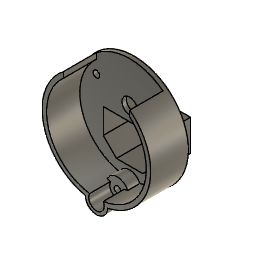
ElementCover v7 (Autodesk Fusion 360 design; units mm, degrees)
Autodesk Fusion 360 part; units mm, degrees
sketch "Sketch1" plane through (0, 0, 0) normal (0, 1, 0) x (1, 0, 0)
  circle A0 centre (-4.2105, -0.0551) radius 22.5
  circle A1 centre (-4.2105, 23.9449) radius 3.5
  circle A2 centre (-4.2105, 23.9449) radius 1.5
  circle A3 centre (-4.2105, -0.0551) radius 24.5
  circle A4 centre (-4.2105, 23.9449) radius 5
  line L0 (-19.2105, -24.5551) -> (10.7895, -24.5551)
  line L1 (10.7895, -24.5551) -> (10.7895, -11.0151)
  line L2 (10.7895, -11.0151) -> (-19.2105, -11.0151)
  line L3 (-19.2105, -11.0151) -> (-19.2105, -24.5551)
  circle A5 centre (-19.2105, -11.0151) radius 1.5
  circle A6 centre (-19.2105, -11.0151) radius 3
  circle A7 centre (10.7895, -11.0151) radius 1.5
  circle A8 centre (10.7895, -11.0151) radius 3
  line L4 (10.7895, -24.5551) -> (-4.2105, -24.5551)
  line L5 (-4.2105, -24.5551) -> (-4.2105, -16.8301)
  line L6 (-4.2105, -16.8301) -> (10.7895, -16.8301)
  line L7 (10.7895, -16.8301) -> (10.7895, -24.5551)
  line L8 (-4.2105, 22.4449) -> (-4.2105, 17.4449)
  line L9 (-4.2105, 17.4449) -> (7.7395, 17.4449)
  line L10 (7.7395, 17.4449) -> (7.7395, 0.1449)
  line L11 (7.7395, 0.1449) -> (-4.2105, 0.1449)
  line L12 (-4.2105, 0.1449) -> (-4.2105, 17.4449)
  line L13 (-4.2105, 17.4449) -> (-16.1605, 17.4449)
  line L14 (-16.1605, 17.4449) -> (-16.1605, 0.1449)
  line L15 (-16.1605, 0.1449) -> (-4.2105, 0.1449)
  line L16 (-4.2105, 0.1449) -> (-4.2105, 17.4449)
  line L17 (7.7395, 17.4449) -> (1.7395, 17.4449)
  line L18 (1.7395, 17.4449) -> (1.7395, 11.4449)
  line L19 (1.7395, 11.4449) -> (7.7395, 11.4449)
  line L20 (7.7395, 11.4449) -> (7.7395, 17.4449)
  line L21 (-16.1605, 17.4449) -> (-10.1605, 17.4449)
  line L22 (-10.1605, 17.4449) -> (-10.1605, 11.4449)
  line L23 (-10.1605, 11.4449) -> (-16.1605, 11.4449)
  line L24 (-16.1605, 11.4449) -> (-16.1605, 17.4449)
  line L25 (-10.1605, 17.4449) -> (-16.1605, 11.4449)
  line L26 (7.7395, 11.4449) -> (1.7395, 17.4449)
  line L27 (-4.2105, -0.0551) -> (-4.2105, -24.5551)
  line L28 (-4.2105, -0.0551) -> (-4.2105, 22.4449)
  line L29 (-4.2105, 22.4449) -> (-4.2105, 24.4449)
  circle A9 centre (-4.2105, -6.0151) radius 3.5
  line L30 (-4.2105, -11.0151) -> (-4.2105, -6.0151)
  line L31 (-4.2105, 23.9449) -> (-4.2105, 22.4449)
  circle A10 centre (-4.2105, 23.9449) radius 3.5
  dimension "d1" = 45
  dimension "d4" = 3
  dimension "d5" = 49
  dimension "d6" = 10
  dimension "d8" = 30
  dimension "d14" = 3
  dimension "d15" = 6
  dimension "d16" = 3
  dimension "d17" = 6
  dimension "d18" = 15
  dimension "d19" = 7.725
  dimension "d22" = 5
  dimension "d23" = 11.95
  dimension "d24" = 17.3
  dimension "d25" = 11.95
  dimension "d26" = 17.3
  dimension "d27" = 6
  dimension "d28" = 6
  dimension "d29" = 6
  dimension "d30" = 6
  dimension "d32" = 7
  dimension "d33" = 7
  dimension "d34" = 5
  dimension "d41" = 7
  dimension "d45" = 13.5401
  constraint concentric A1 A2
  constraint concentric A0 A3
  constraint concentric A2 A4
  constraint horizontal L0
  constraint vertical L1
  constraint horizontal L2
  constraint vertical L3
  constraint tangent A3 L0
  constraint concentric A5 A6
  constraint concentric A7 A8
  constraint horizontal L4
  constraint vertical L5
  constraint horizontal L6
  constraint vertical L7
  constraint coincident A0 L8.start
  constraint vertical L8
  constraint horizontal L9
  constraint vertical L10
  constraint horizontal L11
  constraint vertical L12
  constraint horizontal L13
  constraint vertical L14
  constraint horizontal L15
  constraint vertical L16
  constraint horizontal L17
  constraint vertical L18
  constraint horizontal L19
  constraint vertical L20
  constraint horizontal L21
  constraint vertical L22
  constraint horizontal L23
  constraint vertical L24
  constraint coincident A0.centre A3.centre
  constraint perpendicular L6 L27
  constraint perpendicular L13 L28
  constraint coincident L2.end L3.start
  constraint coincident L1.end L2.start
  constraint coincident A3 L29.end
  constraint parallel L28 L29
  constraint coincident L27 A9.centre
  constraint midpoint L2 L30.start
  constraint coincident A9.centre L30.end
  constraint perpendicular L2 L30
  constraint coincident A1.centre A2.centre
  constraint coincident A2 L8.start
  constraint vertical L31
  constraint coincident L8.start L28.end
  measures "d1" diameter of A0
  measures "d4" diameter of A2
  measures "d5" diameter of A3
  measures "d6" diameter of A4
  measures "d8" distance of L0.start L0.end
  measures "d14" diameter of A5
  measures "d15" diameter of A6
  measures "d16" diameter of A7
  measures "d17" diameter of A8
  measures "d18" distance of L0.end L4.end
  measures "d19" distance of L0.end L6.end
  measures "d22" distance of L8.start L8.end
  measures "d23" distance of L8.end L9.end
  measures "d24" distance of L8.end L11.end
  measures "d25" distance of L8.end L13.end
  measures "d26" distance of L8.end L11.end
  measures "d27" distance of L9.end L17.end
  measures "d28" distance of L9.end L19.end
  measures "d29" distance of L13.end L21.end
  measures "d30" distance of L13.end L23.end
  measures "d32" diameter of A1
  measures "d33" diameter of A9
  measures "d34" distance of A9.centre L30.start
  measures "d41" diameter of A10
  measures "d45" distance of L0.start L2.end
extrude "Extrude1" add sketch "Sketch1" along normal blind 2 contours A0 A4 L1 L2 A8 L8 L9 L10 L11 L17 L20 L27 L28 A9 L30 | A0 A3 A4 L1 L7 | A0 A1 A4 L8 L28 A10 | A0 A1 A3 A4 A10 | A0 A3 L1 L5 L7 L27 | L1 L2 A8 L6 L27 | A0 L5 L6 L27 | A0 A1 L8 L28 A10 | A0 A1 A2 A3 A10 | A0 A4 L2 L3 A6 L8 L13 L14 L15 L21 L24 L27 L28 A9 L30 | A0 A1 A4 L8 L28 A10 | A1 A3 A4 A10 | A0 A3 L3 L5 L27 | A0 L2 L3 A6 L5 L27 | L1 L2 A7 A8 | L1 L2 A7 A8 | A0 A1 L8 L28 A10 | A0 A1 A2 A3 A10 | A0 A1 A3 A4 A10 | A0 A3 A4 L3 | A1 A2 A3 A10 | L9 L10 L17 L20 L26 | L13 L14 L21 L24 L25 | L2 L3 A5 A6 | L2 L3 A5 A6
extrude "Extrude2" add sketch "Sketch1" against normal blind 15 contours A0 A3 A4 L1 L7 | A0 A1 A3 A4 A10 | A1 A3 A4 A10 | A0 A1 A3 A4 A10 | A0 A3 A4 L3
extrude "Extrude3" cut sketch "Sketch1" along normal up to surface (2 mm away) contours L1 L2 A7 | L1 L2 A7 | L2 L3 A5 | L2 L3 A5
extrude "Extrude4" add sketch "Sketch1" against normal blind 5.5 contours A0 A1 A4 L8 L28 A10 | A0 A1 L8 L28 A10 | A0 A1 A2 A3 A10 | A0 A1 A4 L8 L28 A10 | A0 A1 L8 L28 A10 | A0 A1 A2 A3 A10 | A1 A2 A3 A10
extrude "Extrude5" cut sketch "Sketch1" along normal blind 2 contours A0 A1 L8 L28 A10 | A0 A1 A2 A3 A10 | A0 A1 L8 L28 A10 | A0 A1 A2 A3 A10 | A1 A2 A3 A10
extrude "Extrude6" cut sketch "Sketch1" against normal blind 3 contours A0 A1 L8 L28 A10 | A0 A1 A2 A3 A10 | A0 A1 L8 L28 A10 | A0 A1 A2 A3 A10 | A1 A2 A3 A10
sketch "Sketch3" plane through (0, 2, 0) normal (0, 1, 0) x (-1, 0, 0)
  circle A0 centre (4.2105, -23.9449) radius 3.5
  line L0 (-7.7395, -11.4449) -> (-7.7395, -0.1449)
  line L1 (-7.7395, -0.1449) -> (16.1605, -0.1449)
  line L2 (16.1605, -0.1449) -> (16.1605, -11.4449)
  line L3 (16.1605, -11.4449) -> (10.1605, -17.4449)
  line L4 (10.1605, -17.4449) -> (-1.7395, -17.4449)
  line L5 (-1.7395, -17.4449) -> (-7.7395, -11.4449)
  circle A1 centre (19.2105, 11.0151) radius 1.5
  circle A2 centre (4.2105, 6.0151) radius 3.5
  circle A3 centre (-10.7895, 11.0151) radius 1.5
  arc A4 (-0.7895, -23.9292) -> (9.2105, -23.9292) centre (4.2105, -23.9449) ccw
  arc A5 (9.2105, -23.9292) -> (-0.7895, -23.9292) centre (4.2105, 0.0551) ccw
  line L6 (18.1605, -12.2733) -> (10.9889, -19.4449)
  line L7 (10.9889, -19.4449) -> (-2.5679, -19.4449)
  line L8 (-2.5679, -19.4449) -> (-9.7395, -12.2733)
  line L9 (-9.7395, -12.2733) -> (-9.7395, 1.8551)
  line L10 (-9.7395, 1.8551) -> (18.1605, 1.8551)
  line L11 (18.1605, 1.8551) -> (18.1605, -12.2733)
  dimension "d42" = -2
extrude "Extrude7" add sketch "Sketch3" along normal blind 11.5 contours L6 L7 L8 L9 L10 L11
equation "d19 = ( 15.45 / 2 ) * 1 mm"
equation "d23 = ( 23.9 / 2 ) * 1 mm"
